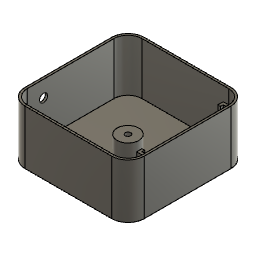
lightAutomationPrototype v1 (Autodesk Fusion 360 design; units mm, degrees)
Autodesk Fusion 360 part; units mm, degrees
sketch "Sketch1" plane through (0, 0, 0) normal (0, 1, 0) x (1, 0, 0)
  line L0 (30, 0) -> (190, 0)
  line L1 (220, -30) -> (220, -190)
  line L2 (190, -220) -> (30, -220)
  line L3 (0, -190) -> (0, -30)
  arc A0 (30, 0) -> (0, -30) centre (30, -30) ccw
  arc A1 (220, -30) -> (190, 0) centre (190, -30) ccw
  arc A2 (0, -190) -> (30, -220) centre (30, -190) ccw
  arc A3 (190, -220) -> (220, -190) centre (190, -190) ccw
  arc A4 (30, -4) -> (4, -30) centre (30, -30) ccw
  line L4 (4, -190) -> (4, -30)
  arc A5 (4, -190) -> (30, -216) centre (30, -190) ccw
  line L5 (190, -216) -> (30, -216)
  arc A6 (190, -216) -> (216, -190) centre (190, -190) ccw
  line L6 (216, -30) -> (216, -190)
  arc A7 (216, -30) -> (190, -4) centre (190, -30) ccw
  line L7 (30, -4) -> (190, -4)
  line L8 (30, -30) -> (190, -190) construction
  line L9 (30, -190) -> (190, -30) construction
  circle A8 centre (110, -110) radius 20
  point P0 (220, 0)
  point P1 (0, -220)
  dimension "d3" = 220
  dimension "d4" = 220
  dimension "d5" = 30
  dimension "d6" = 30
  dimension "d7" = 30
  dimension "d9" = 4
  dimension "d14" = 40
  constraint horizontal L0
  constraint vertical L1
  constraint horizontal L2
  constraint vertical L3
  constraint coincident origin L3
  constraint coincident origin L0
  constraint tangent L3 A0
  constraint tangent L0 A0
  constraint coincident P0 L0
  constraint coincident P0 L1
  constraint tangent L0 A1
  constraint tangent L1 A1
  constraint coincident P1 L2
  constraint coincident P1 L3
  constraint tangent L2 A2
  constraint tangent L3 A2
  constraint equal A1 A2
  constraint tangent L2 A3
  constraint tangent L1 A3
  constraint coincident A0.centre A4.centre
  constraint coincident A3.centre A6.centre
  constraint coincident A2.centre A5.centre
  constraint coincident A1.centre A7.centre
  constraint midpoint L9 A8.centre
  measures "d3" distance of origin P0
  measures "d4" distance of origin P1
  measures "d5" radius of A0
  measures "d6" radius of A1 P0
  measures "d7" radius of A3
  measures "d14" diameter of A8
extrude "Extrude2" add sketch "Sketch1" along normal blind 4 contours A4 L4 A5 L5 A6 L6 A7 L7 makes body 1
extrude "Extrude1" add sketch "Sketch1" along normal blind 100 separate body contours L0 L1 L2 L3 A0 A1 A2 A3 makes body 2
extrude "Extrude3" add sketch "Sketch1" along normal blind 40 contours A8 bodies 1
hole "Hole2" at (110, 0, 110) direction (0, 1, 0) diameter 33.526 depth 30 tip angle 180 bodies 1
thread "Thread2" "ISO Metric profile 35.0 M35x1.5 6H"
hole "Hole3" at (110, 40, 110) direction (0, -1, 0) diameter 10 depth 10 tip angle 180 bodies 1
sketch "Sketch3" plane through (216, 0, 0) normal (-1, 0, 0) x (0, 0, 1)
  line L0 (30, 0) -> (190, 0)
  line L1 (190, 0) -> (190, 100)
  line L2 (190, 100) -> (30, 100)
  line L3 (30, 100) -> (30, 0)
  line L4 (30, 0) -> (40, 0)
  line L5 (40, 0) -> (40, 100)
  line L6 (40, 100) -> (30, 100)
  line L7 (30, 100) -> (30, 0)
  line L8 (190, 0) -> (180, 0)
  line L9 (180, 0) -> (180, 100)
  line L10 (180, 100) -> (190, 100)
  line L11 (190, 100) -> (190, 0)
  dimension "d29" = 10
  dimension "d30" = 10
  constraint horizontal L4
  constraint vertical L5
  constraint horizontal L6
  constraint vertical L7
  constraint coincident L0.start L3.end
  constraint horizontal L8
  constraint vertical L9
  constraint horizontal L10
  constraint vertical L11
  constraint coincident L0.end L1.start
  measures "d29" distance of L0.start L4.end
  measures "d30" distance of L0.end L8.end
extrude "Extrude1'" add sketch "Sketch3" along normal blind 10 separate body contours L0 L2 L3 L4 L5 L6 L7 | L0 L1 L2 L8 L9 L10 L11 makes body 3 at (212.6667, 66.6667, 30) makes body 4 at (216, 66.6667, 183.3333) in component "circuitBoard"
sketch "Sketch4" plane through (0, 100, 0) normal (0, 1, 0) x (-1, 0, 0)
  line L0 (-216, 40) -> (-216, 30)
  line L1 (-216, 30) -> (-206, 30)
  line L2 (-206, 30) -> (-206, 40)
  line L3 (-206, 40) -> (-216, 40)
  line L4 (-216, 40) -> (-211, 40)
  line L5 (-211, 40) -> (-211, 35)
  line L6 (-211, 35) -> (-216, 35)
  line L7 (-216, 35) -> (-216, 40)
  constraint horizontal L4
  constraint vertical L5
  constraint horizontal L6
  constraint vertical L7
  constraint coincident L0.start L3.end
sketch "Sketch5" plane through (0, 100, 0) normal (0, 1, 0) x (-1, 0, 0)
  line L0 (-216, 190) -> (-216, 180)
  line L1 (-216, 180) -> (-206, 180)
  line L2 (-206, 180) -> (-206, 190)
  line L3 (-206, 190) -> (-216, 190)
  line L4 (-216, 180) -> (-211, 180)
  line L5 (-211, 180) -> (-211, 185)
  line L6 (-211, 185) -> (-216, 185)
  line L7 (-216, 185) -> (-216, 180)
  dimension "d33" = 5
  dimension "d34" = 5
  constraint horizontal L4
  constraint vertical L5
  constraint horizontal L6
  constraint vertical L7
  constraint coincident L0.end L1.start
  measures "d33" distance of L0.end L4.end
  measures "d34" distance of L0.end L6.end
extrude "Extrude2'" cut sketch "Sketch4" sketch "Sketch5" against normal blind 96 contours L0 L3 L4 L5 L6 L7 of sketch 2 contours L0 L1 L4 L5 L6 L7 bodies 3 4 in component "circuitBoard"
sketch "Sketch6" plane through (0, 0, 0) normal (-1, 0, 0) x (0, 0, 1)
  line L0 (30, 0) -> (190, 0)
  line L1 (190, 0) -> (190, 100)
  line L2 (190, 100) -> (30, 100)
  line L3 (30, 100) -> (30, 0)
  point P0 (160, 70)
  dimension "d39" = 30
  dimension "d40" = 30
  measures "d39" distance of L2 P0
  measures "d40" distance of L1 P0
hole "Hole4" at (0, 70, 160) direction (1, 0, 0) diameter 15 depth 10 tip angle 180 bodies 2
component "circuitBoard" placed x (1, 0, 0) y (0, 1, 0) z (0, 0, 1) at (0, 0, 0)
equation "side = 220 mm" comment "length of sides"
equation "for = 30 mm" comment "fillet outer radius"
equation "d3 = side"
equation "d4 = side"
equation "d5 = for"
equation "d6 = for"
equation "d7 = for"
equation "t = 4 mm" comment "thickness of object"
equation "d9 = t"
equation "h = 100 mm" comment "height of object"
equation "d11 = h"
equation "br = 40 mm" comment "bulb radius"
equation "d14 = br"
equation "d15 = t"
equation "bsl = 40 mm" comment "bulb screw length"
equation "d18 = bsl"
equation "d35 = -h + t"
equation "wes = 30 mm" comment "wire entry side"
equation "wet = 30 mm" comment "wire entry top"
equation "d39 = wet"
equation "d40 = wes"
